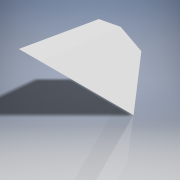
# Autodesk Inventor part: FrontTriangularJoist
Saved by Autodesk Inventor 2018 (Build 220112000, 112)
## iProperties
Created: 2018-07-21
Part Number: FrontTriangularJoist
Material: Generic
Document SubType Name: Modeling
Designer: jjsch
Density: 1 g/cm^3
Appearance: Default
Author: jjsch
Autodesk Inventor part; units mm, degrees
ref_plane "YZ Plane" through (0, 0, 0) normal (1, 0, 0) x (0, 1, 0)
ref_plane "XZ Plane" through (0, 0, 0) normal (0, 1, 0) x (-1, 0, 0)
ref_plane "XY Plane" through (0, 0, 0) normal (0, 0, 1) x (1, 0, 0)
sketch "Sketch1" plane through (0, 0, 0) normal (1, 0, 0) x (0, 1, 0)
  line L0 (0, 0) -> (215.5261, 215.5261)
  line L1 (0, 0) -> (304.8, 0) construction
  line L2 (215.5261, 215.5261) -> (278.3879, 152.6644)
  line L3 (278.3879, 152.6644) -> (62.8618, -62.8618)
  line L4 (62.8618, -62.8618) -> (0, 0)
  line L5 (125.7236, 0) -> (0, 0)
  line L6 (215.5261, 215.5261) -> (215.5261, 89.8026)
  dimension "d0" = 304.8
  dimension "d1" = 45
  dimension "d2" = 88.9
  constraints: 14 end point, 4 perpendicular, 2 horizontal, 2 point on line, 1 equal length
  measures "d0" distance of L0.start L0.end
  measures "d1" angle of L1 L0
  measures "d2" distance of L0.end L2.end
extrude "Extrusion1" add sketch "Sketch1" along normal blind 38.1 contours L0 L6 L3 L5
body "Solid1"
